Autodesk Fusion 360 part; units mm, degrees
(part 2 of 12)
  arc A499 (36.5761, 84.6112) -> (39.1161, 84.6112) centre (37.8461, 84.6112) ccw
  arc A500 (36.5761, 84.6112) -> (39.1161, 84.6112) centre (37.8461, 84.6112) ccw
  arc A501 (39.1161, 84.6112) -> (36.5761, 84.6112) centre (37.8461, 84.6112) ccw
  arc A502 (75.4661, 87.1512) -> (72.9261, 87.1512) centre (74.1961, 87.1512) ccw
  arc A503 (72.9261, 87.1512) -> (75.4661, 87.1512) centre (74.1961, 87.1512) ccw
  arc A504 (75.4661, 87.1512) -> (72.9261, 87.1512) centre (74.1961, 87.1512) ccw
  arc A505 (72.9261, 87.1512) -> (75.4661, 87.1512) centre (74.1961, 87.1512) ccw
  arc A506 (72.9261, 87.1512) -> (75.4661, 87.1512) centre (74.1961, 87.1512) ccw
  arc A507 (75.4661, 87.1512) -> (72.9261, 87.1512) centre (74.1961, 87.1512) ccw
  arc A508 (66.5761, 84.6112) -> (69.1161, 84.6112) centre (67.8461, 84.6112) ccw
  arc A509 (69.1161, 84.6112) -> (66.5761, 84.6112) centre (67.8461, 84.6112) ccw
  arc A510 (69.1161, 84.6112) -> (66.5761, 84.6112) centre (67.8461, 84.6112) ccw
  arc A511 (66.5761, 84.6112) -> (69.1161, 84.6112) centre (67.8461, 84.6112) ccw
  arc A512 (66.5761, 84.6112) -> (69.1161, 84.6112) centre (67.8461, 84.6112) ccw
  arc A513 (69.1161, 84.6112) -> (66.5761, 84.6112) centre (67.8461, 84.6112) ccw
  arc A514 (105.4661, 87.1512) -> (102.9261, 87.1512) centre (104.1961, 87.1512) ccw
  arc A515 (102.9261, 87.1512) -> (105.4661, 87.1512) centre (104.1961, 87.1512) ccw
  arc A516 (105.4661, 87.1512) -> (102.9261, 87.1512) centre (104.1961, 87.1512) ccw
  arc A517 (102.9261, 87.1512) -> (105.4661, 87.1512) centre (104.1961, 87.1512) ccw
  arc A518 (102.9261, 87.1512) -> (105.4661, 87.1512) centre (104.1961, 87.1512) ccw
  arc A519 (105.4661, 87.1512) -> (102.9261, 87.1512) centre (104.1961, 87.1512) ccw
  arc A520 (96.5761, 84.6112) -> (99.1161, 84.6112) centre (97.8461, 84.6112) ccw
  arc A521 (99.1161, 84.6112) -> (96.5761, 84.6112) centre (97.8461, 84.6112) ccw
  arc A522 (96.5761, 84.6112) -> (99.1161, 84.6112) centre (97.8461, 84.6112) ccw
  arc A523 (99.1161, 84.6112) -> (96.5761, 84.6112) centre (97.8461, 84.6112) ccw
  arc A524 (99.1161, 84.6112) -> (96.5761, 84.6112) centre (97.8461, 84.6112) ccw
  arc A525 (96.5761, 84.6112) -> (99.1161, 84.6112) centre (97.8461, 84.6112) ccw
  arc A526 (135.4661, 87.1512) -> (132.9261, 87.1512) centre (134.1961, 87.1512) ccw
  arc A527 (132.9261, 87.1512) -> (135.4661, 87.1512) centre (134.1961, 87.1512) ccw
  arc A528 (135.4661, 87.1512) -> (132.9261, 87.1512) centre (134.1961, 87.1512) ccw
  arc A529 (132.9261, 87.1512) -> (135.4661, 87.1512) centre (134.1961, 87.1512) ccw
  arc A530 (135.4661, 87.1512) -> (132.9261, 87.1512) centre (134.1961, 87.1512) ccw
  arc A531 (132.9261, 87.1512) -> (135.4661, 87.1512) centre (134.1961, 87.1512) ccw
  arc A532 (129.1161, 84.6112) -> (126.5761, 84.6112) centre (127.8461, 84.6112) ccw
  arc A533 (126.5761, 84.6112) -> (129.1161, 84.6112) centre (127.8461, 84.6112) ccw
  arc A534 (129.1161, 84.6112) -> (126.5761, 84.6112) centre (127.8461, 84.6112) ccw
  arc A535 (126.5761, 84.6112) -> (129.1161, 84.6112) centre (127.8461, 84.6112) ccw
  arc A536 (126.5761, 84.6112) -> (129.1161, 84.6112) centre (127.8461, 84.6112) ccw
  arc A537 (129.1161, 84.6112) -> (126.5761, 84.6112) centre (127.8461, 84.6112) ccw
  arc A538 (162.9261, 87.1512) -> (165.4661, 87.1512) centre (164.1961, 87.1512) ccw
  arc A539 (165.4661, 87.1512) -> (162.9261, 87.1512) centre (164.1961, 87.1512) ccw
  arc A540 (162.9261, 87.1512) -> (165.4661, 87.1512) centre (164.1961, 87.1512) ccw
  arc A541 (165.4661, 87.1512) -> (162.9261, 87.1512) centre (164.1961, 87.1512) ccw
  arc A542 (165.4661, 87.1512) -> (162.9261, 87.1512) centre (164.1961, 87.1512) ccw
  arc A543 (162.9261, 87.1512) -> (165.4661, 87.1512) centre (164.1961, 87.1512) ccw
  arc A544 (159.1161, 84.6112) -> (156.5761, 84.6112) centre (157.8461, 84.6112) ccw
  arc A545 (156.5761, 84.6112) -> (159.1161, 84.6112) centre (157.8461, 84.6112) ccw
  arc A546 (159.1161, 84.6112) -> (156.5761, 84.6112) centre (157.8461, 84.6112) ccw
  arc A547 (156.5761, 84.6112) -> (159.1161, 84.6112) centre (157.8461, 84.6112) ccw
  arc A548 (156.5761, 84.6112) -> (159.1161, 84.6112) centre (157.8461, 84.6112) ccw
  arc A549 (159.1161, 84.6112) -> (156.5761, 84.6112) centre (157.8461, 84.6112) ccw
  arc A550 (192.9261, 87.1512) -> (195.4661, 87.1512) centre (194.1961, 87.1512) ccw
  arc A551 (195.4661, 87.1512) -> (192.9261, 87.1512) centre (194.1961, 87.1512) ccw
  arc A552 (192.9261, 87.1512) -> (195.4661, 87.1512) centre (194.1961, 87.1512) ccw
  arc A553 (195.4661, 87.1512) -> (192.9261, 87.1512) centre (194.1961, 87.1512) ccw
  arc A554 (195.4661, 87.1512) -> (192.9261, 87.1512) centre (194.1961, 87.1512) ccw
  arc A555 (192.9261, 87.1512) -> (195.4661, 87.1512) centre (194.1961, 87.1512) ccw
  arc A556 (186.5761, 84.6112) -> (189.1161, 84.6112) centre (187.8461, 84.6112) ccw
  arc A557 (189.1161, 84.6112) -> (186.5761, 84.6112) centre (187.8461, 84.6112) ccw
  arc A558 (186.5761, 84.6112) -> (189.1161, 84.6112) centre (187.8461, 84.6112) ccw
  arc A559 (189.1161, 84.6112) -> (186.5761, 84.6112) centre (187.8461, 84.6112) ccw
  arc A560 (186.5761, 84.6112) -> (189.1161, 84.6112) centre (187.8461, 84.6112) ccw
  arc A561 (189.1161, 84.6112) -> (186.5761, 84.6112) centre (187.8461, 84.6112) ccw
  arc A562 (222.9261, 87.1512) -> (225.4661, 87.1512) centre (224.1961, 87.1512) ccw
  arc A563 (225.4661, 87.1512) -> (222.9261, 87.1512) centre (224.1961, 87.1512) ccw
  arc A564 (222.9261, 87.1512) -> (225.4661, 87.1512) centre (224.1961, 87.1512) ccw
  arc A565 (225.4661, 87.1512) -> (222.9261, 87.1512) centre (224.1961, 87.1512) ccw
  arc A566 (225.4661, 87.1512) -> (222.9261, 87.1512) centre (224.1961, 87.1512) ccw
  arc A567 (222.9261, 87.1512) -> (225.4661, 87.1512) centre (224.1961, 87.1512) ccw
  arc A568 (219.1161, 84.6112) -> (216.5761, 84.6112) centre (217.8461, 84.6112) ccw
  arc A569 (216.5761, 84.6112) -> (219.1161, 84.6112) centre (217.8461, 84.6112) ccw
  arc A570 (219.1161, 84.6112) -> (216.5761, 84.6112) centre (217.8461, 84.6112) ccw
  arc A571 (216.5761, 84.6112) -> (219.1161, 84.6112) centre (217.8461, 84.6112) ccw
  arc A572 (219.1161, 84.6112) -> (216.5761, 84.6112) centre (217.8461, 84.6112) ccw
  arc A573 (216.5761, 84.6112) -> (219.1161, 84.6112) centre (217.8461, 84.6112) ccw
  arc A574 (45.4661, 57.1512) -> (42.9261, 57.1512) centre (44.1961, 57.1512) ccw
  arc A575 (42.9261, 57.1512) -> (45.4661, 57.1512) centre (44.1961, 57.1512) ccw
  arc A576 (42.9261, 57.1512) -> (45.4661, 57.1512) centre (44.1961, 57.1512) ccw
  arc A577 (45.4661, 57.1512) -> (42.9261, 57.1512) centre (44.1961, 57.1512) ccw
  arc A578 (42.9261, 57.1512) -> (45.4661, 57.1512) centre (44.1961, 57.1512) ccw
  arc A579 (45.4661, 57.1512) -> (42.9261, 57.1512) centre (44.1961, 57.1512) ccw
  arc A580 (39.1161, 54.6112) -> (36.5761, 54.6112) centre (37.8461, 54.6112) ccw
  arc A581 (36.5761, 54.6112) -> (39.1161, 54.6112) centre (37.8461, 54.6112) ccw
  arc A582 (36.5761, 54.6112) -> (39.1161, 54.6112) centre (37.8461, 54.6112) ccw
  arc A583 (39.1161, 54.6112) -> (36.5761, 54.6112) centre (37.8461, 54.6112) ccw
  arc A584 (39.1161, 54.6112) -> (36.5761, 54.6112) centre (37.8461, 54.6112) ccw
  arc A585 (36.5761, 54.6112) -> (39.1161, 54.6112) centre (37.8461, 54.6112) ccw
  arc A586 (72.9261, 57.1512) -> (75.4661, 57.1512) centre (74.1961, 57.1512) ccw
  arc A587 (75.4661, 57.1512) -> (72.9261, 57.1512) centre (74.1961, 57.1512) ccw
  arc A588 (75.4661, 57.1512) -> (72.9261, 57.1512) centre (74.1961, 57.1512) ccw
  arc A589 (72.9261, 57.1512) -> (75.4661, 57.1512) centre (74.1961, 57.1512) ccw
  arc A590 (72.9261, 57.1512) -> (75.4661, 57.1512) centre (74.1961, 57.1512) ccw
  arc A591 (75.4661, 57.1512) -> (72.9261, 57.1512) centre (74.1961, 57.1512) ccw
  arc A592 (66.5761, 54.6112) -> (69.1161, 54.6112) centre (67.8461, 54.6112) ccw
  arc A593 (69.1161, 54.6112) -> (66.5761, 54.6112) centre (67.8461, 54.6112) ccw
  arc A594 (66.5761, 54.6112) -> (69.1161, 54.6112) centre (67.8461, 54.6112) ccw
  arc A595 (69.1161, 54.6112) -> (66.5761, 54.6112) centre (67.8461, 54.6112) ccw
  arc A596 (69.1161, 54.6112) -> (66.5761, 54.6112) centre (67.8461, 54.6112) ccw
  arc A597 (66.5761, 54.6112) -> (69.1161, 54.6112) centre (67.8461, 54.6112) ccw
  arc A598 (102.9261, 57.1512) -> (105.4661, 57.1512) centre (104.1961, 57.1512) ccw
  arc A599 (105.4661, 57.1512) -> (102.9261, 57.1512) centre (104.1961, 57.1512) ccw
  arc A600 (105.4661, 57.1512) -> (102.9261, 57.1512) centre (104.1961, 57.1512) ccw
  arc A601 (102.9261, 57.1512) -> (105.4661, 57.1512) centre (104.1961, 57.1512) ccw
  arc A602 (102.9261, 57.1512) -> (105.4661, 57.1512) centre (104.1961, 57.1512) ccw
  arc A603 (105.4661, 57.1512) -> (102.9261, 57.1512) centre (104.1961, 57.1512) ccw
  arc A604 (96.5761, 54.6112) -> (99.1161, 54.6112) centre (97.8461, 54.6112) ccw
  arc A605 (99.1161, 54.6112) -> (96.5761, 54.6112) centre (97.8461, 54.6112) ccw
  arc A606 (96.5761, 54.6112) -> (99.1161, 54.6112) centre (97.8461, 54.6112) ccw
  arc A607 (99.1161, 54.6112) -> (96.5761, 54.6112) centre (97.8461, 54.6112) ccw
  arc A608 (99.1161, 54.6112) -> (96.5761, 54.6112) centre (97.8461, 54.6112) ccw
  arc A609 (96.5761, 54.6112) -> (99.1161, 54.6112) centre (97.8461, 54.6112) ccw
  arc A610 (135.4661, 57.1512) -> (132.9261, 57.1512) centre (134.1961, 57.1512) ccw
  arc A611 (132.9261, 57.1512) -> (135.4661, 57.1512) centre (134.1961, 57.1512) ccw
  arc A612 (135.4661, 57.1512) -> (132.9261, 57.1512) centre (134.1961, 57.1512) ccw
  arc A613 (132.9261, 57.1512) -> (135.4661, 57.1512) centre (134.1961, 57.1512) ccw
  arc A614 (135.4661, 57.1512) -> (132.9261, 57.1512) centre (134.1961, 57.1512) ccw
  arc A615 (132.9261, 57.1512) -> (135.4661, 57.1512) centre (134.1961, 57.1512) ccw
  arc A616 (126.5761, 54.6112) -> (129.1161, 54.6112) centre (127.8461, 54.6112) ccw
  arc A617 (129.1161, 54.6112) -> (126.5761, 54.6112) centre (127.8461, 54.6112) ccw
  arc A618 (129.1161, 54.6112) -> (126.5761, 54.6112) centre (127.8461, 54.6112) ccw
  arc A619 (126.5761, 54.6112) -> (129.1161, 54.6112) centre (127.8461, 54.6112) ccw
  arc A620 (129.1161, 54.6112) -> (126.5761, 54.6112) centre (127.8461, 54.6112) ccw
  arc A621 (126.5761, 54.6112) -> (129.1161, 54.6112) centre (127.8461, 54.6112) ccw
  arc A622 (165.4661, 57.1512) -> (162.9261, 57.1512) centre (164.1961, 57.1512) ccw
  arc A623 (162.9261, 57.1512) -> (165.4661, 57.1512) centre (164.1961, 57.1512) ccw
  arc A624 (165.4661, 57.1512) -> (162.9261, 57.1512) centre (164.1961, 57.1512) ccw
  arc A625 (162.9261, 57.1512) -> (165.4661, 57.1512) centre (164.1961, 57.1512) ccw
  arc A626 (165.4661, 57.1512) -> (162.9261, 57.1512) centre (164.1961, 57.1512) ccw
  arc A627 (162.9261, 57.1512) -> (165.4661, 57.1512) centre (164.1961, 57.1512) ccw
  arc A628 (156.5761, 54.6112) -> (159.1161, 54.6112) centre (157.8461, 54.6112) ccw
  arc A629 (159.1161, 54.6112) -> (156.5761, 54.6112) centre (157.8461, 54.6112) ccw
  arc A630 (156.5761, 54.6112) -> (159.1161, 54.6112) centre (157.8461, 54.6112) ccw
  arc A631 (159.1161, 54.6112) -> (156.5761, 54.6112) centre (157.8461, 54.6112) ccw
  arc A632 (156.5761, 54.6112) -> (159.1161, 54.6112) centre (157.8461, 54.6112) ccw
  arc A633 (159.1161, 54.6112) -> (156.5761, 54.6112) centre (157.8461, 54.6112) ccw
  arc A634 (195.4661, 57.1512) -> (192.9261, 57.1512) centre (194.1961, 57.1512) ccw
  arc A635 (192.9261, 57.1512) -> (195.4661, 57.1512) centre (194.1961, 57.1512) ccw
  arc A636 (195.4661, 57.1512) -> (192.9261, 57.1512) centre (194.1961, 57.1512) ccw
  arc A637 (192.9261, 57.1512) -> (195.4661, 57.1512) centre (194.1961, 57.1512) ccw
  arc A638 (195.4661, 57.1512) -> (192.9261, 57.1512) centre (194.1961, 57.1512) ccw
  arc A639 (192.9261, 57.1512) -> (195.4661, 57.1512) centre (194.1961, 57.1512) ccw
  arc A640 (186.5761, 54.6112) -> (189.1161, 54.6112) centre (187.8461, 54.6112) ccw
  arc A641 (189.1161, 54.6112) -> (186.5761, 54.6112) centre (187.8461, 54.6112) ccw
  arc A642 (189.1161, 54.6112) -> (186.5761, 54.6112) centre (187.8461, 54.6112) ccw
  arc A643 (186.5761, 54.6112) -> (189.1161, 54.6112) centre (187.8461, 54.6112) ccw
  arc A644 (189.1161, 54.6112) -> (186.5761, 54.6112) centre (187.8461, 54.6112) ccw
  arc A645 (186.5761, 54.6112) -> (189.1161, 54.6112) centre (187.8461, 54.6112) ccw
  arc A646 (225.4661, 57.1512) -> (222.9261, 57.1512) centre (224.1961, 57.1512) ccw
  arc A647 (222.9261, 57.1512) -> (225.4661, 57.1512) centre (224.1961, 57.1512) ccw
  arc A648 (222.9261, 57.1512) -> (225.4661, 57.1512) centre (224.1961, 57.1512) ccw
  arc A649 (225.4661, 57.1512) -> (222.9261, 57.1512) centre (224.1961, 57.1512) ccw
  arc A650 (222.9261, 57.1512) -> (225.4661, 57.1512) centre (224.1961, 57.1512) ccw
  arc A651 (225.4661, 57.1512) -> (222.9261, 57.1512) centre (224.1961, 57.1512) ccw
  arc A652 (219.1161, 54.6112) -> (216.5761, 54.6112) centre (217.8461, 54.6112) ccw
  arc A653 (216.5761, 54.6112) -> (219.1161, 54.6112) centre (217.8461, 54.6112) ccw
  arc A654 (219.1161, 54.6112) -> (216.5761, 54.6112) centre (217.8461, 54.6112) ccw
  arc A655 (216.5761, 54.6112) -> (219.1161, 54.6112) centre (217.8461, 54.6112) ccw
  arc A656 (219.1161, 54.6112) -> (216.5761, 54.6112) centre (217.8461, 54.6112) ccw
  arc A657 (216.5761, 54.6112) -> (219.1161, 54.6112) centre (217.8461, 54.6112) ccw
  arc A658 (45.4661, 27.1512) -> (42.9261, 27.1512) centre (44.1961, 27.1512) ccw
  arc A659 (42.9261, 27.1512) -> (45.4661, 27.1512) centre (44.1961, 27.1512) ccw
  arc A660 (45.4661, 27.1512) -> (42.9261, 27.1512) centre (44.1961, 27.1512) ccw
  arc A661 (42.9261, 27.1512) -> (45.4661, 27.1512) centre (44.1961, 27.1512) ccw
  arc A662 (42.9261, 27.1512) -> (45.4661, 27.1512) centre (44.1961, 27.1512) ccw
  arc A663 (45.4661, 27.1512) -> (42.9261, 27.1512) centre (44.1961, 27.1512) ccw
  arc A664 (36.5761, 24.6112) -> (39.1161, 24.6112) centre (37.8461, 24.6112) ccw
  arc A665 (39.1161, 24.6112) -> (36.5761, 24.6112) centre (37.8461, 24.6112) ccw
  arc A666 (36.5761, 24.6112) -> (39.1161, 24.6112) centre (37.8461, 24.6112) ccw
  arc A667 (39.1161, 24.6112) -> (36.5761, 24.6112) centre (37.8461, 24.6112) ccw
  arc A668 (36.5761, 24.6112) -> (39.1161, 24.6112) centre (37.8461, 24.6112) ccw
  arc A669 (39.1161, 24.6112) -> (36.5761, 24.6112) centre (37.8461, 24.6112) ccw
  arc A670 (81.5494, 27.2071) -> (79.0094, 27.2071) centre (80.2794, 27.2071) ccw
  arc A671 (79.0094, 27.2071) -> (81.5494, 27.2071) centre (80.2794, 27.2071) ccw
  arc A672 (79.0094, 27.2071) -> (81.5494, 27.2071) centre (80.2794, 27.2071) ccw
  arc A673 (81.5494, 27.2071) -> (79.0094, 27.2071) centre (80.2794, 27.2071) ccw
  arc A674 (81.5494, 27.2071) -> (79.0094, 27.2071) centre (80.2794, 27.2071) ccw
  arc A675 (79.0094, 27.2071) -> (81.5494, 27.2071) centre (80.2794, 27.2071) ccw
  arc A676 (75.1994, 24.6671) -> (72.6594, 24.6671) centre (73.9294, 24.6671) ccw
  arc A677 (72.6594, 24.6671) -> (75.1994, 24.6671) centre (73.9294, 24.6671) ccw
  arc A678 (75.1994, 24.6671) -> (72.6594, 24.6671) centre (73.9294, 24.6671) ccw
  arc A679 (72.6594, 24.6671) -> (75.1994, 24.6671) centre (73.9294, 24.6671) ccw
  arc A680 (72.6594, 24.6671) -> (75.1994, 24.6671) centre (73.9294, 24.6671) ccw
  arc A681 (75.1994, 24.6671) -> (72.6594, 24.6671) centre (73.9294, 24.6671) ccw
  arc A682 (109.0094, 27.2071) -> (111.5494, 27.2071) centre (110.2794, 27.2071) ccw
  arc A683 (111.5494, 27.2071) -> (109.0094, 27.2071) centre (110.2794, 27.2071) ccw
  arc A684 (111.5494, 27.2071) -> (109.0094, 27.2071) centre (110.2794, 27.2071) ccw
  arc A685 (109.0094, 27.2071) -> (111.5494, 27.2071) centre (110.2794, 27.2071) ccw
  arc A686 (109.0094, 27.2071) -> (111.5494, 27.2071) centre (110.2794, 27.2071) ccw
  arc A687 (111.5494, 27.2071) -> (109.0094, 27.2071) centre (110.2794, 27.2071) ccw
  arc A688 (102.6594, 24.6671) -> (105.1994, 24.6671) centre (103.9294, 24.6671) ccw
  arc A689 (105.1994, 24.6671) -> (102.6594, 24.6671) centre (103.9294, 24.6671) ccw
  arc A690 (105.1994, 24.6671) -> (102.6594, 24.6671) centre (103.9294, 24.6671) ccw
  arc A691 (102.6594, 24.6671) -> (105.1994, 24.6671) centre (103.9294, 24.6671) ccw
  arc A692 (105.1994, 24.6671) -> (102.6594, 24.6671) centre (103.9294, 24.6671) ccw
  arc A693 (102.6594, 24.6671) -> (105.1994, 24.6671) centre (103.9294, 24.6671) ccw
  arc A694 (139.0094, 27.2071) -> (141.5494, 27.2071) centre (140.2794, 27.2071) ccw
  arc A695 (141.5494, 27.2071) -> (139.0094, 27.2071) centre (140.2794, 27.2071) ccw
  arc A696 (139.0094, 27.2071) -> (141.5494, 27.2071) centre (140.2794, 27.2071) ccw
  arc A697 (141.5494, 27.2071) -> (139.0094, 27.2071) centre (140.2794, 27.2071) ccw
  arc A698 (141.5494, 27.2071) -> (139.0094, 27.2071) centre (140.2794, 27.2071) ccw
  arc A699 (139.0094, 27.2071) -> (141.5494, 27.2071) centre (140.2794, 27.2071) ccw
  arc A700 (135.1994, 24.6671) -> (132.6594, 24.6671) centre (133.9294, 24.6671) ccw
  arc A701 (132.6594, 24.6671) -> (135.1994, 24.6671) centre (133.9294, 24.6671) ccw
  arc A702 (132.6594, 24.6671) -> (135.1994, 24.6671) centre (133.9294, 24.6671) ccw
  arc A703 (135.1994, 24.6671) -> (132.6594, 24.6671) centre (133.9294, 24.6671) ccw
  arc A704 (132.6594, 24.6671) -> (135.1994, 24.6671) centre (133.9294, 24.6671) ccw
  arc A705 (135.1994, 24.6671) -> (132.6594, 24.6671) centre (133.9294, 24.6671) ccw
  arc A706 (169.0094, 27.2071) -> (171.5494, 27.2071) centre (170.2794, 27.2071) ccw
  arc A707 (171.5494, 27.2071) -> (169.0094, 27.2071) centre (170.2794, 27.2071) ccw
  arc A708 (169.0094, 27.2071) -> (171.5494, 27.2071) centre (170.2794, 27.2071) ccw
  arc A709 (171.5494, 27.2071) -> (169.0094, 27.2071) centre (170.2794, 27.2071) ccw
  arc A710 (171.5494, 27.2071) -> (169.0094, 27.2071) centre (170.2794, 27.2071) ccw
  arc A711 (169.0094, 27.2071) -> (171.5494, 27.2071) centre (170.2794, 27.2071) ccw
  arc A712 (162.6594, 24.6671) -> (165.1994, 24.6671) centre (163.9294, 24.6671) ccw
  arc A713 (165.1994, 24.6671) -> (162.6594, 24.6671) centre (163.9294, 24.6671) ccw
  arc A714 (162.6594, 24.6671) -> (165.1994, 24.6671) centre (163.9294, 24.6671) ccw
  arc A715 (165.1994, 24.6671) -> (162.6594, 24.6671) centre (163.9294, 24.6671) ccw
  arc A716 (162.6594, 24.6671) -> (165.1994, 24.6671) centre (163.9294, 24.6671) ccw
  arc A717 (165.1994, 24.6671) -> (162.6594, 24.6671) centre (163.9294, 24.6671) ccw
  arc A718 (199.0094, 27.2071) -> (201.5494, 27.2071) centre (200.2794, 27.2071) ccw
  arc A719 (201.5494, 27.2071) -> (199.0094, 27.2071) centre (200.2794, 27.2071) ccw
  arc A720 (201.5494, 27.2071) -> (199.0094, 27.2071) centre (200.2794, 27.2071) ccw
  arc A721 (199.0094, 27.2071) -> (201.5494, 27.2071) centre (200.2794, 27.2071) ccw
  arc A722 (199.0094, 27.2071) -> (201.5494, 27.2071) centre (200.2794, 27.2071) ccw
  arc A723 (201.5494, 27.2071) -> (199.0094, 27.2071) centre (200.2794, 27.2071) ccw
  arc A724 (195.1994, 24.6671) -> (192.6594, 24.6671) centre (193.9294, 24.6671) ccw
  arc A725 (192.6594, 24.6671) -> (195.1994, 24.6671) centre (193.9294, 24.6671) ccw
  arc A726 (195.1994, 24.6671) -> (192.6594, 24.6671) centre (193.9294, 24.6671) ccw
  arc A727 (192.6594, 24.6671) -> (195.1994, 24.6671) centre (193.9294, 24.6671) ccw
  arc A728 (192.6594, 24.6671) -> (195.1994, 24.6671) centre (193.9294, 24.6671) ccw
  arc A729 (195.1994, 24.6671) -> (192.6594, 24.6671) centre (193.9294, 24.6671) ccw
  arc A730 (120.2692, -60.2389) -> (117.7292, -60.2389) centre (118.9992, -60.2389) ccw
  arc A731 (117.7292, -60.2389) -> (120.2692, -60.2389) centre (118.9992, -60.2389) ccw
  arc A732 (117.7292, -60.2389) -> (120.2692, -60.2389) centre (118.9992, -60.2389) ccw
  arc A733 (120.2692, -60.2389) -> (117.7292, -60.2389) centre (118.9992, -60.2389) ccw
  arc A734 (120.2692, -60.2389) -> (117.7292, -60.2389) centre (118.9992, -60.2389) ccw
  arc A735 (117.7292, -60.2389) -> (120.2692, -60.2389) centre (118.9992, -60.2389) ccw
  arc A736 (113.9192, -62.7789) -> (111.3792, -62.7789) centre (112.6492, -62.7789) ccw
  arc A737 (111.3792, -62.7789) -> (113.9192, -62.7789) centre (112.6492, -62.7789) ccw
  arc A738 (111.3792, -62.7789) -> (113.9192, -62.7789) centre (112.6492, -62.7789) ccw
  arc A739 (113.9192, -62.7789) -> (111.3792, -62.7789) centre (112.6492, -62.7789) ccw
  arc A740 (111.3792, -62.7789) -> (113.9192, -62.7789) centre (112.6492, -62.7789) ccw
  arc A741 (113.9192, -62.7789) -> (111.3792, -62.7789) centre (112.6492, -62.7789) ccw
  arc A742 (42.9261, -2.8488) -> (45.4661, -2.8488) centre (44.1961, -2.8488) ccw
  arc A743 (45.4661, -2.8488) -> (42.9261, -2.8488) centre (44.1961, -2.8488) ccw
  arc A744 (42.9261, -2.8488) -> (45.4661, -2.8488) centre (44.1961, -2.8488) ccw
  arc A745 (45.4661, -2.8488) -> (42.9261, -2.8488) centre (44.1961, -2.8488) ccw
  arc A746 (45.4661, -2.8488) -> (42.9261, -2.8488) centre (44.1961, -2.8488) ccw
  arc A747 (42.9261, -2.8488) -> (45.4661, -2.8488) centre (44.1961, -2.8488) ccw
  arc A748 (39.1161, -5.3888) -> (36.5761, -5.3888) centre (37.8461, -5.3888) ccw
  arc A749 (36.5761, -5.3888) -> (39.1161, -5.3888) centre (37.8461, -5.3888) ccw
  arc A750 (39.1161, -5.3888) -> (36.5761, -5.3888) centre (37.8461, -5.3888) ccw
  arc A751 (36.5761, -5.3888) -> (39.1161, -5.3888) centre (37.8461, -5.3888) ccw
  arc A752 (39.1161, -5.3888) -> (36.5761, -5.3888) centre (37.8461, -5.3888) ccw
  arc A753 (36.5761, -5.3888) -> (39.1161, -5.3888) centre (37.8461, -5.3888) ccw
  arc A754 (89.9314, -2.8919) -> (92.4714, -2.8919) centre (91.2014, -2.8919) ccw
  arc A755 (92.4714, -2.8919) -> (89.9314, -2.8919) centre (91.2014, -2.8919) ccw
  arc A756 (92.4714, -2.8919) -> (89.9314, -2.8919) centre (91.2014, -2.8919) ccw
  arc A757 (89.9314, -2.8919) -> (92.4714, -2.8919) centre (91.2014, -2.8919) ccw
  arc A758 (89.9314, -2.8919) -> (92.4714, -2.8919) centre (91.2014, -2.8919) ccw
  arc A759 (92.4714, -2.8919) -> (89.9314, -2.8919) centre (91.2014, -2.8919) ccw
  arc A760 (86.1214, -5.432) -> (83.5814, -5.432) centre (84.8514, -5.432) ccw
  arc A761 (83.5814, -5.432) -> (86.1214, -5.432) centre (84.8514, -5.432) ccw
  arc A762 (83.5814, -5.432) -> (86.1214, -5.432) centre (84.8514, -5.432) ccw
  arc A763 (86.1214, -5.432) -> (83.5814, -5.432) centre (84.8514, -5.432) ccw
  arc A764 (83.5814, -5.432) -> (86.1214, -5.432) centre (84.8514, -5.432) ccw
  arc A765 (86.1214, -5.432) -> (83.5814, -5.432) centre (84.8514, -5.432) ccw
  arc A766 (122.4714, -2.8919) -> (119.9314, -2.8919) centre (121.2014, -2.8919) ccw
  arc A767 (119.9314, -2.8919) -> (122.4714, -2.8919) centre (121.2014, -2.8919) ccw
  arc A768 (122.4714, -2.8919) -> (119.9314, -2.8919) centre (121.2014, -2.8919) ccw
  arc A769 (119.9314, -2.8919) -> (122.4714, -2.8919) centre (121.2014, -2.8919) ccw
  arc A770 (119.9314, -2.8919) -> (122.4714, -2.8919) centre (121.2014, -2.8919) ccw
  arc A771 (122.4714, -2.8919) -> (119.9314, -2.8919) centre (121.2014, -2.8919) ccw
  arc A772 (116.1214, -5.432) -> (113.5814, -5.432) centre (114.8514, -5.432) ccw
  arc A773 (113.5814, -5.432) -> (116.1214, -5.432) centre (114.8514, -5.432) ccw
  arc A774 (116.1214, -5.432) -> (113.5814, -5.432) centre (114.8514, -5.432) ccw
  arc A775 (113.5814, -5.432) -> (116.1214, -5.432) centre (114.8514, -5.432) ccw
  arc A776 (113.5814, -5.432) -> (116.1214, -5.432) centre (114.8514, -5.432) ccw
  arc A777 (116.1214, -5.432) -> (113.5814, -5.432) centre (114.8514, -5.432) ccw
  arc A778 (149.9314, -2.8919) -> (152.4714, -2.8919) centre (151.2014, -2.8919) ccw
  arc A779 (152.4714, -2.8919) -> (149.9314, -2.8919) centre (151.2014, -2.8919) ccw
  arc A780 (149.9314, -2.8919) -> (152.4714, -2.8919) centre (151.2014, -2.8919) ccw
  arc A781 (152.4714, -2.8919) -> (149.9314, -2.8919) centre (151.2014, -2.8919) ccw
  arc A782 (149.9314, -2.8919) -> (152.4714, -2.8919) centre (151.2014, -2.8919) ccw
  arc A783 (152.4714, -2.8919) -> (149.9314, -2.8919) centre (151.2014, -2.8919) ccw
  arc A784 (146.1214, -5.432) -> (143.5814, -5.432) centre (144.8514, -5.432) ccw
  arc A785 (143.5814, -5.432) -> (146.1214, -5.432) centre (144.8514, -5.432) ccw
  arc A786 (146.1214, -5.432) -> (143.5814, -5.432) centre (144.8514, -5.432) ccw
  arc A787 (143.5814, -5.432) -> (146.1214, -5.432) centre (144.8514, -5.432) ccw
  arc A788 (143.5814, -5.432) -> (146.1214, -5.432) centre (144.8514, -5.432) ccw
  arc A789 (146.1214, -5.432) -> (143.5814, -5.432) centre (144.8514, -5.432) ccw
  arc A790 (182.4714, -2.8919) -> (179.9314, -2.8919) centre (181.2014, -2.8919) ccw
  arc A791 (179.9314, -2.8919) -> (182.4714, -2.8919) centre (181.2014, -2.8919) ccw
  arc A792 (179.9314, -2.8919) -> (182.4714, -2.8919) centre (181.2014, -2.8919) ccw
  arc A793 (182.4714, -2.8919) -> (179.9314, -2.8919) centre (181.2014, -2.8919) ccw
  arc A794 (182.4714, -2.8919) -> (179.9314, -2.8919) centre (181.2014, -2.8919) ccw
  arc A795 (179.9314, -2.8919) -> (182.4714, -2.8919) centre (181.2014, -2.8919) ccw
  arc A796 (176.1214, -5.432) -> (173.5814, -5.432) centre (174.8514, -5.432) ccw
  arc A797 (173.5814, -5.432) -> (176.1214, -5.432) centre (174.8514, -5.432) ccw
  arc A798 (176.1214, -5.432) -> (173.5814, -5.432) centre (174.8514, -5.432) ccw
  arc A799 (173.5814, -5.432) -> (176.1214, -5.432) centre (174.8514, -5.432) ccw
  arc A800 (173.5814, -5.432) -> (176.1214, -5.432) centre (174.8514, -5.432) ccw
  arc A801 (176.1214, -5.432) -> (173.5814, -5.432) centre (174.8514, -5.432) ccw
  arc A802 (209.9314, -2.8919) -> (212.4714, -2.8919) centre (211.2014, -2.8919) ccw
  arc A803 (212.4714, -2.8919) -> (209.9314, -2.8919) centre (211.2014, -2.8919) ccw
  arc A804 (212.4714, -2.8919) -> (209.9314, -2.8919) centre (211.2014, -2.8919) ccw
  arc A805 (209.9314, -2.8919) -> (212.4714, -2.8919) centre (211.2014, -2.8919) ccw
  arc A806 (212.4714, -2.8919) -> (209.9314, -2.8919) centre (211.2014, -2.8919) ccw
  arc A807 (209.9314, -2.8919) -> (212.4714, -2.8919) centre (211.2014, -2.8919) ccw
  arc A808 (203.5814, -5.432) -> (206.1214, -5.432) centre (204.8514, -5.432) ccw
  arc A809 (206.1214, -5.432) -> (203.5814, -5.432) centre (204.8514, -5.432) ccw
  arc A810 (206.1214, -5.432) -> (203.5814, -5.432) centre (204.8514, -5.432) ccw
  arc A811 (203.5814, -5.432) -> (206.1214, -5.432) centre (204.8514, -5.432) ccw
  arc A812 (206.1214, -5.432) -> (203.5814, -5.432) centre (204.8514, -5.432) ccw
  arc A813 (203.5814, -5.432) -> (206.1214, -5.432) centre (204.8514, -5.432) ccw
  arc A814 (161.7983, -60.2389) -> (164.3383, -60.2389) centre (163.0683, -60.2389) ccw
  arc A815 (164.3383, -60.2389) -> (161.7983, -60.2389) centre (163.0683, -60.2389) ccw
  arc A816 (164.3383, -60.2389) -> (161.7983, -60.2389) centre (163.0683, -60.2389) ccw
  arc A817 (161.7983, -60.2389) -> (164.3383, -60.2389) centre (163.0683, -60.2389) ccw
  arc A818 (161.7983, -60.2389) -> (164.3383, -60.2389) centre (163.0683, -60.2389) ccw
  arc A819 (164.3383, -60.2389) -> (161.7983, -60.2389) centre (163.0683, -60.2389) ccw
  arc A820 (155.4483, -62.7789) -> (157.9883, -62.7789) centre (156.7183, -62.7789) ccw
  arc A821 (157.9883, -62.7789) -> (155.4483, -62.7789) centre (156.7183, -62.7789) ccw
  arc A822 (155.4483, -62.7789) -> (157.9883, -62.7789) centre (156.7183, -62.7789) ccw
  arc A823 (157.9883, -62.7789) -> (155.4483, -62.7789) centre (156.7183, -62.7789) ccw
  arc A824 (155.4483, -62.7789) -> (157.9883, -62.7789) centre (156.7183, -62.7789) ccw
  arc A825 (157.9883, -62.7789) -> (155.4483, -62.7789) centre (156.7183, -62.7789) ccw
  arc A826 (42.9261, -32.8488) -> (45.4661, -32.8488) centre (44.1961, -32.8488) ccw
  arc A827 (45.4661, -32.8488) -> (42.9261, -32.8488) centre (44.1961, -32.8488) ccw
  arc A828 (45.4661, -32.8488) -> (42.9261, -32.8488) centre (44.1961, -32.8488) ccw
  arc A829 (42.9261, -32.8488) -> (45.4661, -32.8488) centre (44.1961, -32.8488) ccw
  arc A830 (45.4661, -32.8488) -> (42.9261, -32.8488) centre (44.1961, -32.8488) ccw
  arc A831 (42.9261, -32.8488) -> (45.4661, -32.8488) centre (44.1961, -32.8488) ccw
  arc A832 (39.1161, -35.3888) -> (36.5761, -35.3888) centre (37.8461, -35.3888) ccw
  arc A833 (36.5761, -35.3888) -> (39.1161, -35.3888) centre (37.8461, -35.3888) ccw
  arc A834 (39.1161, -35.3888) -> (36.5761, -35.3888) centre (37.8461, -35.3888) ccw
  arc A835 (36.5761, -35.3888) -> (39.1161, -35.3888) centre (37.8461, -35.3888) ccw
  arc A836 (36.5761, -35.3888) -> (39.1161, -35.3888) centre (37.8461, -35.3888) ccw
  arc A837 (39.1161, -35.3888) -> (36.5761, -35.3888) centre (37.8461, -35.3888) ccw
  arc A838 (99.4564, -32.864) -> (101.9964, -32.864) centre (100.7264, -32.864) ccw
  arc A839 (101.9964, -32.864) -> (99.4564, -32.864) centre (100.7264, -32.864) ccw
  arc A840 (99.4564, -32.864) -> (101.9964, -32.864) centre (100.7264, -32.864) ccw
  arc A841 (101.9964, -32.864) -> (99.4564, -32.864) centre (100.7264, -32.864) ccw
  arc A842 (101.9964, -32.864) -> (99.4564, -32.864) centre (100.7264, -32.864) ccw
  arc A843 (99.4564, -32.864) -> (101.9964, -32.864) centre (100.7264, -32.864) ccw
  arc A844 (93.1064, -35.404) -> (95.6464, -35.404) centre (94.3764, -35.404) ccw
  arc A845 (95.6464, -35.404) -> (93.1064, -35.404) centre (94.3764, -35.404) ccw
  arc A846 (95.6464, -35.404) -> (93.1064, -35.404) centre (94.3764, -35.404) ccw
  arc A847 (93.1064, -35.404) -> (95.6464, -35.404) centre (94.3764, -35.404) ccw
  arc A848 (95.6464, -35.404) -> (93.1064, -35.404) centre (94.3764, -35.404) ccw
  arc A849 (93.1064, -35.404) -> (95.6464, -35.404) centre (94.3764, -35.404) ccw
  arc A850 (18.681, -44.6179) -> (20.181, -44.6179) centre (19.431, -44.6179) ccw
  arc A851 (20.181, -44.6179) -> (18.681, -44.6179) centre (19.431, -44.6179) ccw
  arc A852 (20.181, -44.6179) -> (18.681, -44.6179) centre (19.431, -44.6179) ccw
  arc A853 (18.681, -44.6179) -> (20.181, -44.6179) centre (19.431, -44.6179) ccw
  arc A854 (20.181, -44.6179) -> (18.681, -44.6179) centre (19.431, -44.6179) ccw
  arc A855 (18.681, -44.6179) -> (20.181, -44.6179) centre (19.431, -44.6179) ccw
  arc A856 (18.681, -42.0779) -> (20.181, -42.0779) centre (19.431, -42.0779) ccw
  arc A857 (20.181, -42.0779) -> (18.681, -42.0779) centre (19.431, -42.0779) ccw
  arc A858 (20.181, -42.0779) -> (18.681, -42.0779) centre (19.431, -42.0779) ccw
  arc A859 (18.681, -42.0779) -> (20.181, -42.0779) centre (19.431, -42.0779) ccw
  arc A860 (20.181, -42.0779) -> (18.681, -42.0779) centre (19.431, -42.0779) ccw
  arc A861 (18.681, -42.0779) -> (20.181, -42.0779) centre (19.431, -42.0779) ccw
  arc A862 (20.181, -39.5379) -> (18.681, -39.5379) centre (19.431, -39.5379) ccw
  arc A863 (18.681, -39.5379) -> (20.181, -39.5379) centre (19.431, -39.5379) ccw
  arc A864 (18.681, -39.5379) -> (20.181, -39.5379) centre (19.431, -39.5379) ccw
  arc A865 (20.181, -39.5379) -> (18.681, -39.5379) centre (19.431, -39.5379) ccw
  arc A866 (20.181, -39.5379) -> (18.681, -39.5379) centre (19.431, -39.5379) ccw
  arc A867 (18.681, -39.5379) -> (20.181, -39.5379) centre (19.431, -39.5379) ccw
  arc A868 (20.181, -36.9979) -> (18.681, -36.9979) centre (19.431, -36.9979) ccw
  arc A869 (18.681, -36.9979) -> (20.181, -36.9979) centre (19.431, -36.9979) ccw
  arc A870 (18.681, -36.9979) -> (20.181, -36.9979) centre (19.431, -36.9979) ccw
  arc A871 (20.181, -36.9979) -> (18.681, -36.9979) centre (19.431, -36.9979) ccw
  arc A872 (18.681, -36.9979) -> (20.181, -36.9979) centre (19.431, -36.9979) ccw
  arc A873 (20.181, -36.9979) -> (18.681, -36.9979) centre (19.431, -36.9979) ccw
  arc A874 (18.681, -34.4579) -> (20.181, -34.4579) centre (19.431, -34.4579) ccw
  arc A875 (20.181, -34.4579) -> (18.681, -34.4579) centre (19.431, -34.4579) ccw
  arc A876 (18.681, -34.4579) -> (20.181, -34.4579) centre (19.431, -34.4579) ccw
  arc A877 (20.181, -34.4579) -> (18.681, -34.4579) centre (19.431, -34.4579) ccw
  arc A878 (20.181, -34.4579) -> (18.681, -34.4579) centre (19.431, -34.4579) ccw
  arc A879 (18.681, -34.4579) -> (20.181, -34.4579) centre (19.431, -34.4579) ccw
  arc A880 (18.681, -31.9179) -> (20.181, -31.9179) centre (19.431, -31.9179) ccw
  arc A881 (20.181, -31.9179) -> (18.681, -31.9179) centre (19.431, -31.9179) ccw
  arc A882 (18.681, -31.9179) -> (20.181, -31.9179) centre (19.431, -31.9179) ccw
  arc A883 (20.181, -31.9179) -> (18.681, -31.9179) centre (19.431, -31.9179) ccw
  arc A884 (18.681, -31.9179) -> (20.181, -31.9179) centre (19.431, -31.9179) ccw
  arc A885 (20.181, -31.9179) -> (18.681, -31.9179) centre (19.431, -31.9179) ccw
  arc A886 (18.681, -29.3779) -> (20.181, -29.3779) centre (19.431, -29.3779) ccw
  arc A887 (20.181, -29.3779) -> (18.681, -29.3779) centre (19.431, -29.3779) ccw
  arc A888 (18.681, -29.3779) -> (20.181, -29.3779) centre (19.431, -29.3779) ccw
  arc A889 (20.181, -29.3779) -> (18.681, -29.3779) centre (19.431, -29.3779) ccw
  arc A890 (20.181, -29.3779) -> (18.681, -29.3779) centre (19.431, -29.3779) ccw
  arc A891 (18.681, -29.3779) -> (20.181, -29.3779) centre (19.431, -29.3779) ccw
  arc A892 (18.681, -26.8378) -> (20.181, -26.8378) centre (19.431, -26.8378) ccw
  arc A893 (20.181, -26.8378) -> (18.681, -26.8378) centre (19.431, -26.8378) ccw
  arc A894 (20.181, -26.8378) -> (18.681, -26.8378) centre (19.431, -26.8378) ccw
  arc A895 (18.681, -26.8378) -> (20.181, -26.8378) centre (19.431, -26.8378) ccw
  arc A896 (20.181, -26.8378) -> (18.681, -26.8378) centre (19.431, -26.8378) ccw
  arc A897 (18.681, -26.8378) -> (20.181, -26.8378) centre (19.431, -26.8378) ccw
  arc A898 (20.181, -24.2978) -> (18.681, -24.2978) centre (19.431, -24.2978) ccw
  arc A899 (18.681, -24.2978) -> (20.181, -24.2978) centre (19.431, -24.2978) ccw
  arc A900 (18.681, -24.2978) -> (20.181, -24.2978) centre (19.431, -24.2978) ccw
  arc A901 (20.181, -24.2978) -> (18.681, -24.2978) centre (19.431, -24.2978) ccw
  arc A902 (18.681, -24.2978) -> (20.181, -24.2978) centre (19.431, -24.2978) ccw
  arc A903 (20.181, -24.2978) -> (18.681, -24.2978) centre (19.431, -24.2978) ccw
  arc A904 (20.181, -21.7578) -> (18.681, -21.7578) centre (19.431, -21.7578) ccw
  arc A905 (18.681, -21.7578) -> (20.181, -21.7578) centre (19.431, -21.7578) ccw
  arc A906 (18.681, -21.7578) -> (20.181, -21.7578) centre (19.431, -21.7578) ccw
  arc A907 (20.181, -21.7578) -> (18.681, -21.7578) centre (19.431, -21.7578) ccw
  arc A908 (18.681, -21.7578) -> (20.181, -21.7578) centre (19.431, -21.7578) ccw
  arc A909 (20.181, -21.7578) -> (18.681, -21.7578) centre (19.431, -21.7578) ccw
  arc A910 (18.681, -19.2178) -> (20.181, -19.2178) centre (19.431, -19.2178) ccw
  arc A911 (20.181, -19.2178) -> (18.681, -19.2178) centre (19.431, -19.2178) ccw
  arc A912 (18.681, -19.2178) -> (20.181, -19.2178) centre (19.431, -19.2178) ccw
  arc A913 (20.181, -19.2178) -> (18.681, -19.2178) centre (19.431, -19.2178) ccw
  arc A914 (20.181, -19.2178) -> (18.681, -19.2178) centre (19.431, -19.2178) ccw
  arc A915 (18.681, -19.2178) -> (20.181, -19.2178) centre (19.431, -19.2178) ccw
  arc A916 (20.181, -16.6778) -> (18.681, -16.6778) centre (19.431, -16.6778) ccw
  arc A917 (18.681, -16.6778) -> (20.181, -16.6778) centre (19.431, -16.6778) ccw
  arc A918 (20.181, -16.6778) -> (18.681, -16.6778) centre (19.431, -16.6778) ccw
  arc A919 (18.681, -16.6778) -> (20.181, -16.6778) centre (19.431, -16.6778) ccw
  arc A920 (18.681, -16.6778) -> (20.181, -16.6778) centre (19.431, -16.6778) ccw
  arc A921 (20.181, -16.6778) -> (18.681, -16.6778) centre (19.431, -16.6778) ccw
  arc A922 (20.181, -14.1378) -> (18.681, -14.1378) centre (19.431, -14.1378) ccw
  arc A923 (18.681, -14.1378) -> (20.181, -14.1378) centre (19.431, -14.1378) ccw
  arc A924 (18.681, -14.1378) -> (20.181, -14.1378) centre (19.431, -14.1378) ccw
  arc A925 (20.181, -14.1378) -> (18.681, -14.1378) centre (19.431, -14.1378) ccw
  arc A926 (20.181, -14.1378) -> (18.681, -14.1378) centre (19.431, -14.1378) ccw
  arc A927 (18.681, -14.1378) -> (20.181, -14.1378) centre (19.431, -14.1378) ccw
  arc A928 (20.181, -11.5978) -> (18.681, -11.5978) centre (19.431, -11.5978) ccw
  arc A929 (18.681, -11.5978) -> (20.181, -11.5978) centre (19.431, -11.5978) ccw
  arc A930 (20.181, -11.5978) -> (18.681, -11.5978) centre (19.431, -11.5978) ccw
  arc A931 (18.681, -11.5978) -> (20.181, -11.5978) centre (19.431, -11.5978) ccw
  arc A932 (20.181, -11.5978) -> (18.681, -11.5978) centre (19.431, -11.5978) ccw
  arc A933 (18.681, -11.5978) -> (20.181, -11.5978) centre (19.431, -11.5978) ccw
  arc A934 (12.561, -44.6179) -> (11.061, -44.6179) centre (11.811, -44.6179) ccw
  arc A935 (11.061, -44.6179) -> (12.561, -44.6179) centre (11.811, -44.6179) ccw
  arc A936 (12.561, -44.6179) -> (11.061, -44.6179) centre (11.811, -44.6179) ccw
  arc A937 (11.061, -44.6179) -> (12.561, -44.6179) centre (11.811, -44.6179) ccw
  arc A938 (11.061, -44.6179) -> (12.561, -44.6179) centre (11.811, -44.6179) ccw
  arc A939 (12.561, -44.6179) -> (11.061, -44.6179) centre (11.811, -44.6179) ccw
  arc A940 (11.061, -42.0779) -> (12.561, -42.0779) centre (11.811, -42.0779) ccw
  arc A941 (12.561, -42.0779) -> (11.061, -42.0779) centre (11.811, -42.0779) ccw
  arc A942 (11.061, -42.0779) -> (12.561, -42.0779) centre (11.811, -42.0779) ccw
  arc A943 (12.561, -42.0779) -> (11.061, -42.0779) centre (11.811, -42.0779) ccw
  arc A944 (11.061, -42.0779) -> (12.561, -42.0779) centre (11.811, -42.0779) ccw
  arc A945 (12.561, -42.0779) -> (11.061, -42.0779) centre (11.811, -42.0779) ccw
  arc A946 (12.561, -39.5379) -> (11.061, -39.5379) centre (11.811, -39.5379) ccw
  arc A947 (11.061, -39.5379) -> (12.561, -39.5379) centre (11.811, -39.5379) ccw
  arc A948 (12.561, -39.5379) -> (11.061, -39.5379) centre (11.811, -39.5379) ccw
  arc A949 (11.061, -39.5379) -> (12.561, -39.5379) centre (11.811, -39.5379) ccw
  arc A950 (11.061, -39.5379) -> (12.561, -39.5379) centre (11.811, -39.5379) ccw
  arc A951 (12.561, -39.5379) -> (11.061, -39.5379) centre (11.811, -39.5379) ccw
  arc A952 (12.561, -36.9979) -> (11.061, -36.9979) centre (11.811, -36.9979) ccw
  arc A953 (11.061, -36.9979) -> (12.561, -36.9979) centre (11.811, -36.9979) ccw
  arc A954 (12.561, -36.9979) -> (11.061, -36.9979) centre (11.811, -36.9979) ccw
  arc A955 (11.061, -36.9979) -> (12.561, -36.9979) centre (11.811, -36.9979) ccw
  arc A956 (12.561, -36.9979) -> (11.061, -36.9979) centre (11.811, -36.9979) ccw
  arc A957 (11.061, -36.9979) -> (12.561, -36.9979) centre (11.811, -36.9979) ccw
  arc A958 (11.061, -34.4579) -> (12.561, -34.4579) centre (11.811, -34.4579) ccw
  arc A959 (12.561, -34.4579) -> (11.061, -34.4579) centre (11.811, -34.4579) ccw
  arc A960 (11.061, -34.4579) -> (12.561, -34.4579) centre (11.811, -34.4579) ccw
  arc A961 (12.561, -34.4579) -> (11.061, -34.4579) centre (11.811, -34.4579) ccw
  arc A962 (12.561, -34.4579) -> (11.061, -34.4579) centre (11.811, -34.4579) ccw
  arc A963 (11.061, -34.4579) -> (12.561, -34.4579) centre (11.811, -34.4579) ccw
  arc A964 (11.061, -31.9179) -> (12.561, -31.9179) centre (11.811, -31.9179) ccw
  arc A965 (12.561, -31.9179) -> (11.061, -31.9179) centre (11.811, -31.9179) ccw
  arc A966 (12.561, -31.9179) -> (11.061, -31.9179) centre (11.811, -31.9179) ccw
  arc A967 (11.061, -31.9179) -> (12.561, -31.9179) centre (11.811, -31.9179) ccw
  arc A968 (12.561, -31.9179) -> (11.061, -31.9179) centre (11.811, -31.9179) ccw
  arc A969 (11.061, -31.9179) -> (12.561, -31.9179) centre (11.811, -31.9179) ccw
  arc A970 (12.561, -29.3779) -> (11.061, -29.3779) centre (11.811, -29.3779) ccw
  arc A971 (11.061, -29.3779) -> (12.561, -29.3779) centre (11.811, -29.3779) ccw
  arc A972 (11.061, -29.3779) -> (12.561, -29.3779) centre (11.811, -29.3779) ccw
  arc A973 (12.561, -29.3779) -> (11.061, -29.3779) centre (11.811, -29.3779) ccw
  arc A974 (11.061, -29.3779) -> (12.561, -29.3779) centre (11.811, -29.3779) ccw
  arc A975 (12.561, -29.3779) -> (11.061, -29.3779) centre (11.811, -29.3779) ccw
  arc A976 (12.561, -26.8378) -> (11.061, -26.8378) centre (11.811, -26.8378) ccw
  arc A977 (11.061, -26.8378) -> (12.561, -26.8378) centre (11.811, -26.8378) ccw
  arc A978 (11.061, -26.8378) -> (12.561, -26.8378) centre (11.811, -26.8378) ccw
  arc A979 (12.561, -26.8378) -> (11.061, -26.8378) centre (11.811, -26.8378) ccw
  arc A980 (12.561, -26.8378) -> (11.061, -26.8378) centre (11.811, -26.8378) ccw
  arc A981 (11.061, -26.8378) -> (12.561, -26.8378) centre (11.811, -26.8378) ccw
  arc A982 (12.561, -24.2978) -> (11.061, -24.2978) centre (11.811, -24.2978) ccw
  arc A983 (11.061, -24.2978) -> (12.561, -24.2978) centre (11.811, -24.2978) ccw
  arc A984 (12.561, -24.2978) -> (11.061, -24.2978) centre (11.811, -24.2978) ccw
  arc A985 (11.061, -24.2978) -> (12.561, -24.2978) centre (11.811, -24.2978) ccw
  arc A986 (11.061, -24.2978) -> (12.561, -24.2978) centre (11.811, -24.2978) ccw
  arc A987 (12.561, -24.2978) -> (11.061, -24.2978) centre (11.811, -24.2978) ccw
  arc A988 (12.561, -21.7578) -> (11.061, -21.7578) centre (11.811, -21.7578) ccw
  arc A989 (11.061, -21.7578) -> (12.561, -21.7578) centre (11.811, -21.7578) ccw
  arc A990 (11.061, -21.7578) -> (12.561, -21.7578) centre (11.811, -21.7578) ccw
  arc A991 (12.561, -21.7578) -> (11.061, -21.7578) centre (11.811, -21.7578) ccw
  arc A992 (12.561, -21.7578) -> (11.061, -21.7578) centre (11.811, -21.7578) ccw
  arc A993 (11.061, -21.7578) -> (12.561, -21.7578) centre (11.811, -21.7578) ccw
  arc A994 (11.061, -19.2178) -> (12.561, -19.2178) centre (11.811, -19.2178) ccw
  arc A995 (12.561, -19.2178) -> (11.061, -19.2178) centre (11.811, -19.2178) ccw
  arc A996 (12.561, -19.2178) -> (11.061, -19.2178) centre (11.811, -19.2178) ccw
  arc A997 (11.061, -19.2178) -> (12.561, -19.2178) centre (11.811, -19.2178) ccw
  arc A998 (11.061, -19.2178) -> (12.561, -19.2178) centre (11.811, -19.2178) ccw
  arc A999 (12.561, -19.2178) -> (11.061, -19.2178) centre (11.811, -19.2178) ccw
  arc A1000 (11.061, -16.6778) -> (12.561, -16.6778) centre (11.811, -16.6778) ccw
  arc A1001 (12.561, -16.6778) -> (11.061, -16.6778) centre (11.811, -16.6778) ccw
  arc A1002 (11.061, -16.6778) -> (12.561, -16.6778) centre (11.811, -16.6778) ccw
  arc A1003 (12.561, -16.6778) -> (11.061, -16.6778) centre (11.811, -16.6778) ccw
  arc A1004 (12.561, -16.6778) -> (11.061, -16.6778) centre (11.811, -16.6778) ccw
  arc A1005 (11.061, -16.6778) -> (12.561, -16.6778) centre (11.811, -16.6778) ccw
  arc A1006 (11.061, -14.1378) -> (12.561, -14.1378) centre (11.811, -14.1378) ccw
  arc A1007 (12.561, -14.1378) -> (11.061, -14.1378) centre (11.811, -14.1378) ccw
  arc A1008 (12.561, -14.1378) -> (11.061, -14.1378) centre (11.811, -14.1378) ccw
  arc A1009 (11.061, -14.1378) -> (12.561, -14.1378) centre (11.811, -14.1378) ccw
  arc A1010 (11.061, -14.1378) -> (12.561, -14.1378) centre (11.811, -14.1378) ccw
  arc A1011 (12.561, -14.1378) -> (11.061, -14.1378) centre (11.811, -14.1378) ccw
  line L195 (11.061, -10.8478) -> (12.561, -10.8478)
  line L196 (12.561, -10.8478) -> (12.561, -12.3478)
  line L197 (12.561, -12.3478) -> (11.061, -12.3478)
  line L198 (11.061, -12.3478) -> (11.061, -10.8478)
  line L199 (12.561, -10.8478) -> (12.561, -12.3478)
  line L200 (11.061, -10.8478) -> (12.561, -10.8478)
  line L201 (12.561, -12.3478) -> (11.061, -12.3478)
  line L202 (11.061, -12.3478) -> (11.061, -10.8478)
  line L203 (11.061, -12.3478) -> (11.061, -10.8478)
  line L204 (12.561, -10.8478) -> (12.561, -12.3478)
  line L205 (12.561, -12.3478) -> (11.061, -12.3478)
  line L206 (11.061, -10.8478) -> (12.561, -10.8478)
  arc A1012 (217.4364, 4.7852) -> (218.9364, 4.7852) centre (218.1864, 4.7852) ccw
  arc A1013 (218.9364, 4.7852) -> (217.4364, 4.7852) centre (218.1864, 4.7852) ccw
  arc A1014 (217.4364, 4.7852) -> (218.9364, 4.7852) centre (218.1864, 4.7852) ccw
  arc A1015 (218.9364, 4.7852) -> (217.4364, 4.7852) centre (218.1864, 4.7852) ccw
  arc A1016 (217.4364, 4.7852) -> (218.9364, 4.7852) centre (218.1864, 4.7852) ccw
  arc A1017 (218.9364, 4.7852) -> (217.4364, 4.7852) centre (218.1864, 4.7852) ccw
  arc A1018 (218.9364, 7.3252) -> (217.4364, 7.3252) centre (218.1864, 7.3252) ccw
  arc A1019 (217.4364, 7.3252) -> (218.9364, 7.3252) centre (218.1864, 7.3252) ccw
  arc A1020 (217.4364, 7.3252) -> (218.9364, 7.3252) centre (218.1864, 7.3252) ccw
  arc A1021 (218.9364, 7.3252) -> (217.4364, 7.3252) centre (218.1864, 7.3252) ccw
  arc A1022 (218.9364, 7.3252) -> (217.4364, 7.3252) centre (218.1864, 7.3252) ccw
  arc A1023 (217.4364, 7.3252) -> (218.9364, 7.3252) centre (218.1864, 7.3252) ccw
  arc A1024 (217.4364, 9.8652) -> (218.9364, 9.8652) centre (218.1864, 9.8652) ccw
  arc A1025 (218.9364, 9.8652) -> (217.4364, 9.8652) centre (218.1864, 9.8652) ccw
  arc A1026 (218.9364, 9.8652) -> (217.4364, 9.8652) centre (218.1864, 9.8652) ccw
  arc A1027 (217.4364, 9.8652) -> (218.9364, 9.8652) centre (218.1864, 9.8652) ccw
  arc A1028 (217.4364, 9.8652) -> (218.9364, 9.8652) centre (218.1864, 9.8652) ccw
  arc A1029 (218.9364, 9.8652) -> (217.4364, 9.8652) centre (218.1864, 9.8652) ccw
  arc A1030 (218.9364, 12.4052) -> (217.4364, 12.4052) centre (218.1864, 12.4052) ccw
  arc A1031 (217.4364, 12.4052) -> (218.9364, 12.4052) centre (218.1864, 12.4052) ccw
  arc A1032 (218.9364, 12.4052) -> (217.4364, 12.4052) centre (218.1864, 12.4052) ccw
  arc A1033 (217.4364, 12.4052) -> (218.9364, 12.4052) centre (218.1864, 12.4052) ccw
  arc A1034 (218.9364, 12.4052) -> (217.4364, 12.4052) centre (218.1864, 12.4052) ccw
  arc A1035 (217.4364, 12.4052) -> (218.9364, 12.4052) centre (218.1864, 12.4052) ccw
  arc A1036 (218.9364, 14.9452) -> (217.4364, 14.9452) centre (218.1864, 14.9452) ccw
  arc A1037 (217.4364, 14.9452) -> (218.9364, 14.9452) centre (218.1864, 14.9452) ccw
  arc A1038 (218.9364, 14.9452) -> (217.4364, 14.9452) centre (218.1864, 14.9452) ccw
  arc A1039 (217.4364, 14.9452) -> (218.9364, 14.9452) centre (218.1864, 14.9452) ccw
  arc A1040 (218.9364, 14.9452) -> (217.4364, 14.9452) centre (218.1864, 14.9452) ccw
  arc A1041 (217.4364, 14.9452) -> (218.9364, 14.9452) centre (218.1864, 14.9452) ccw
  arc A1042 (217.4364, 17.4852) -> (218.9364, 17.4852) centre (218.1864, 17.4852) ccw
  arc A1043 (218.9364, 17.4852) -> (217.4364, 17.4852) centre (218.1864, 17.4852) ccw
  arc A1044 (218.9364, 17.4852) -> (217.4364, 17.4852) centre (218.1864, 17.4852) ccw
  arc A1045 (217.4364, 17.4852) -> (218.9364, 17.4852) centre (218.1864, 17.4852) ccw
  arc A1046 (217.4364, 17.4852) -> (218.9364, 17.4852) centre (218.1864, 17.4852) ccw
  arc A1047 (218.9364, 17.4852) -> (217.4364, 17.4852) centre (218.1864, 17.4852) ccw
  arc A1048 (218.9364, 20.0252) -> (217.4364, 20.0252) centre (218.1864, 20.0252) ccw
  arc A1049 (217.4364, 20.0252) -> (218.9364, 20.0252) centre (218.1864, 20.0252) ccw
  arc A1050 (218.9364, 20.0252) -> (217.4364, 20.0252) centre (218.1864, 20.0252) ccw
  arc A1051 (217.4364, 20.0252) -> (218.9364, 20.0252) centre (218.1864, 20.0252) ccw
  arc A1052 (217.4364, 20.0252) -> (218.9364, 20.0252) centre (218.1864, 20.0252) ccw
  arc A1053 (218.9364, 20.0252) -> (217.4364, 20.0252) centre (218.1864, 20.0252) ccw
  arc A1054 (218.9364, 22.5653) -> (217.4364, 22.5653) centre (218.1864, 22.5653) ccw
  arc A1055 (217.4364, 22.5653) -> (218.9364, 22.5653) centre (218.1864, 22.5653) ccw
  arc A1056 (217.4364, 22.5653) -> (218.9364, 22.5653) centre (218.1864, 22.5653) ccw
  arc A1057 (218.9364, 22.5653) -> (217.4364, 22.5653) centre (218.1864, 22.5653) ccw
  arc A1058 (218.9364, 22.5653) -> (217.4364, 22.5653) centre (218.1864, 22.5653) ccw
  arc A1059 (217.4364, 22.5653) -> (218.9364, 22.5653) centre (218.1864, 22.5653) ccw
  arc A1060 (218.9364, 25.1053) -> (217.4364, 25.1053) centre (218.1864, 25.1053) ccw
  arc A1061 (217.4364, 25.1053) -> (218.9364, 25.1053) centre (218.1864, 25.1053) ccw
  arc A1062 (218.9364, 25.1053) -> (217.4364, 25.1053) centre (218.1864, 25.1053) ccw
  arc A1063 (217.4364, 25.1053) -> (218.9364, 25.1053) centre (218.1864, 25.1053) ccw
  arc A1064 (218.9364, 25.1053) -> (217.4364, 25.1053) centre (218.1864, 25.1053) ccw
  arc A1065 (217.4364, 25.1053) -> (218.9364, 25.1053) centre (218.1864, 25.1053) ccw
  arc A1066 (218.9364, 27.6453) -> (217.4364, 27.6453) centre (218.1864, 27.6453) ccw
  arc A1067 (217.4364, 27.6453) -> (218.9364, 27.6453) centre (218.1864, 27.6453) ccw
  arc A1068 (217.4364, 27.6453) -> (218.9364, 27.6453) centre (218.1864, 27.6453) ccw
  arc A1069 (218.9364, 27.6453) -> (217.4364, 27.6453) centre (218.1864, 27.6453) ccw
  arc A1070 (218.9364, 27.6453) -> (217.4364, 27.6453) centre (218.1864, 27.6453) ccw
  arc A1071 (217.4364, 27.6453) -> (218.9364, 27.6453) centre (218.1864, 27.6453) ccw
  arc A1072 (218.9364, 30.1853) -> (217.4364, 30.1853) centre (218.1864, 30.1853) ccw
  arc A1073 (217.4364, 30.1853) -> (218.9364, 30.1853) centre (218.1864, 30.1853) ccw
  arc A1074 (218.9364, 30.1853) -> (217.4364, 30.1853) centre (218.1864, 30.1853) ccw
  arc A1075 (217.4364, 30.1853) -> (218.9364, 30.1853) centre (218.1864, 30.1853) ccw
  arc A1076 (218.9364, 30.1853) -> (217.4364, 30.1853) centre (218.1864, 30.1853) ccw
  arc A1077 (217.4364, 30.1853) -> (218.9364, 30.1853) centre (218.1864, 30.1853) ccw
  arc A1078 (218.9364, 32.7253) -> (217.4364, 32.7253) centre (218.1864, 32.7253) ccw
  arc A1079 (217.4364, 32.7253) -> (218.9364, 32.7253) centre (218.1864, 32.7253) ccw
  arc A1080 (217.4364, 32.7253) -> (218.9364, 32.7253) centre (218.1864, 32.7253) ccw
  arc A1081 (218.9364, 32.7253) -> (217.4364, 32.7253) centre (218.1864, 32.7253) ccw
  arc A1082 (217.4364, 32.7253) -> (218.9364, 32.7253) centre (218.1864, 32.7253) ccw
  arc A1083 (218.9364, 32.7253) -> (217.4364, 32.7253) centre (218.1864, 32.7253) ccw
  arc A1084 (218.9364, 35.2653) -> (217.4364, 35.2653) centre (218.1864, 35.2653) ccw
  arc A1085 (217.4364, 35.2653) -> (218.9364, 35.2653) centre (218.1864, 35.2653) ccw
  arc A1086 (218.9364, 35.2653) -> (217.4364, 35.2653) centre (218.1864, 35.2653) ccw
  arc A1087 (217.4364, 35.2653) -> (218.9364, 35.2653) centre (218.1864, 35.2653) ccw